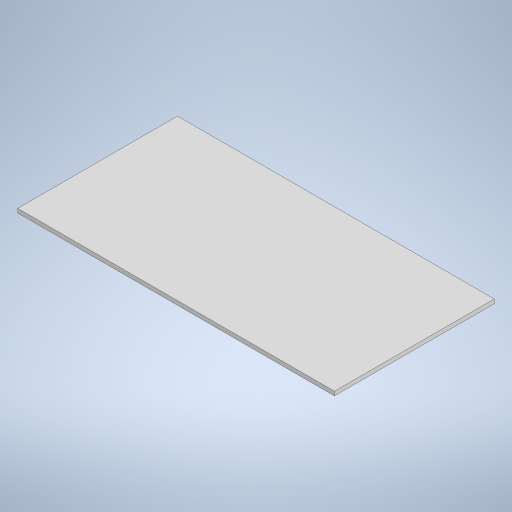
# Autodesk Inventor part: assyBase
Saved by Autodesk Inventor 2023 (Build 270158000, 158)
## iProperties
Created: 2023-06-24
Part Number: assyBase
Material: Generic
Document SubType Name: Modeling
Designer: incep
Density: 1 g/cm^3
Appearance: Default
Author: incep
Autodesk Inventor part; units mm, degrees
ref_plane "YZ Plane" through (0, 0, 0) normal (1, 0, 0) x (0, 1, 0)
ref_plane "XZ Plane" through (0, 0, 0) normal (0, 1, 0) x (-1, 0, 0)
ref_plane "XY Plane" through (0, 0, 0) normal (0, 0, 1) x (1, 0, 0)
sketch "Sketch1" plane through (0, 0, 0) normal (0, 1, 0) x (-1, 0, 0)
  line L0 (387.4, -195.4) -> (-387.4, -195.4)
  line L1 (-387.4, -195.4) -> (-387.4, 195.4)
  line L2 (-387.4, 195.4) -> (387.4, 195.4)
  line L3 (387.4, 195.4) -> (387.4, -195.4)
  point P0 (0, 0)
  point P1 (-387.4, 0)
  point P2 (0, -195.4)
  dimension "d0" = 774.8
  dimension "d1" = 390.8
  constraints: 8 end point, 2 midpoint, 2 parallel, 1 horizontal, 1 horizontal alignment, 1 perpendicular, 1 vertical alignment
  measures "d0" distance of L1.end L2.end
  measures "d1" distance of L0.end L1.end
extrude "Extrusion1" add sketch "Sketch1" along normal blind 10
body "Solid1"
